BatterHolder v3 (Autodesk Fusion 360 design; units mm, degrees)
Autodesk Fusion 360 part; units mm, degrees
note: some values were not read from the file. Chosen so that the rebuilt part matches the saved one: which face or edge a step refers to.
sketch "Sketch1" plane through (0, 0, 0) normal (0, 1, 0) x (1, 0, 0)
  line L0 (0, 0) -> (62, 0)
  line L1 (62, 0) -> (62, -31)
  line L2 (62, -31) -> (0, -31)
  line L3 (0, -31) -> (0, 0)
  dimension "d1" = 62
  dimension "d2" = 31
  constraint horizontal L0
  constraint vertical L1
  constraint horizontal L2
  constraint vertical L3
  constraint coincident L0.start L3.end
  measures "d2" distance of L0.start
extrude "Extrude1" add sketch "Sketch1" along normal blind 15
fillet "Fillet1" radius 1 12 edges at (0, 7.5, 0) (62, 7.5, 0) (31, 0, 0) (31, 15, 0) (62, 7.5, 31) (62, 0, 15.5) (62, 15, 15.5) (0, 7.5, 31) (31, 0, 31) (31, 15, 31) (0, 0, 15.5) (0, 15, 15.5)
